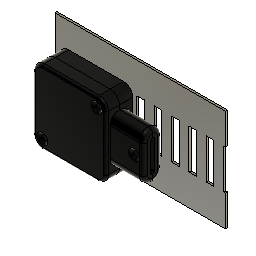
Prog Backpack v22 (Autodesk Fusion 360 design; units mm, degrees)
Autodesk Fusion 360 part; units mm, degrees
sketch "GCP Metal Case" plane through (0, 0, 0) normal (0, 1, 0) x (1, 0, 0)
  line L0 (-58.7401, 16.0721) -> (43.7757, 16.0721) construction
  line L1 (-58.7401, 46.7071) -> (43.7757, 46.7071)
  line L2 (43.7757, -14.5628) -> (-58.7401, -14.5628)
  line L3 (57.6, 4.0721) -> (53.15, 4.0721)
  line L4 (32.25, 4.0721) -> (32.25, 28.0721)
  line L5 (-15.55, 28.0721) -> (-15.55, 4.0721)
  line L6 (-30.45, 16.0721) -> (-26, 16.0721) construction
  line L7 (11.35, 4.0721) -> (11.35, 28.0721)
  line L8 (26.25, 28.0721) -> (26.25, 4.0721)
  line L9 (0.9, 4.0721) -> (0.9, 28.0721)
  line L10 (15.8, 4.0721) -> (11.35, 4.0721)
  line L11 (47.15, 28.0721) -> (47.15, 4.0721)
  line L12 (53.15, 4.0721) -> (53.15, 28.0721)
  line L13 (-9.55, 4.0721) -> (-9.55, 28.0721)
  line L14 (-20, 28.0721) -> (-15.55, 28.0721)
  line L15 (-26, 4.0721) -> (-30.45, 4.0721)
  line L16 (-30.45, 4.0721) -> (-30.45, 28.0721)
  line L17 (21.8, 4.0721) -> (21.8, 28.0721)
  line L18 (5.35, 28.0721) -> (5.35, 4.0721)
  line L19 (-58.7401, -14.5628) -> (-58.7401, 46.7071)
  line L20 (-20, 4.0721) -> (-20, 28.0721)
  line L21 (-5.1, 4.0721) -> (-9.55, 4.0721)
  line L22 (-15.55, 4.0721) -> (-20, 4.0721)
  line L23 (0.9, 28.0721) -> (5.35, 28.0721)
  line L24 (36.7, 28.0721) -> (36.7, 4.0721)
  line L25 (26.25, 4.0721) -> (21.8, 4.0721)
  line L26 (15.8, 28.0721) -> (15.8, 4.0721)
  line L27 (21.8, 28.0721) -> (26.25, 28.0721)
  line L28 (53.15, 28.0721) -> (57.6, 28.0721)
  line L29 (47.15, 4.0721) -> (42.7, 4.0721)
  line L30 (-5.1, 28.0721) -> (-5.1, 4.0721)
  line L31 (-9.55, 28.0721) -> (-5.1, 28.0721)
  line L32 (36.7, 4.0721) -> (32.25, 4.0721)
  line L33 (-30.45, 28.0721) -> (-26, 28.0721)
  line L34 (11.35, 28.0721) -> (15.8, 28.0721)
  line L35 (42.7, 4.0721) -> (42.7, 28.0721)
  line L36 (-26, 28.0721) -> (-26, 4.0721)
  line L37 (5.35, 4.0721) -> (0.9, 4.0721)
  line L38 (43.7757, 46.7071) -> (43.7757, -14.5628)
  line L39 (32.25, 28.0721) -> (36.7, 28.0721)
  line L40 (57.6, 28.0721) -> (57.6, 4.0721)
  line L41 (42.7, 28.0721) -> (47.15, 28.0721)
  dimension "d3" = 10.45
  dimension "d4" = 0
  dimension "d23" = 4.45
  dimension "d24" = 24
  constraint horizontal L1
  constraint vertical L38
  constraint horizontal L2
  constraint vertical L19
  constraint midpoint L0.start L19
  constraint midpoint L0.end L38
  constraint horizontal L33
  constraint vertical L36
  constraint horizontal L15
  constraint vertical L16
  constraint midpoint L6.start L16
  constraint midpoint L6.end L36
  constraint collinear L0 L6
  measures "d23" distance of L16 L36
  measures "d24" distance of L15 L33
extrude "Extrude1" add sketch "GCP Metal Case" along normal blind 1.25 contours L1 L2 L19 L29 L35 L38 L41 makes body 1
sketch "Internals" plane through (0, 0, 0) normal (0, 1, 0) x (1, 0, 0)
  line L0 (-20, 4.0721) -> (-20, 28.0721)
  line L1 (-15.55, 4.0721) -> (-20, 4.0721)
  line L2 (-15.55, 28.0721) -> (-15.55, 4.0721)
  line L3 (-20, 28.0721) -> (-15.55, 28.0721)
  line L4 (-47.05, 3.5721) -> (-31.55, 3.5721)
  line L5 (-31.55, 41.5721) -> (-47.05, 41.5721)
  line L6 (-30.45, 4.0721) -> (-30.45, 28.0721)
  line L7 (-26, 4.0721) -> (-30.45, 4.0721)
  line L8 (-26, 28.0721) -> (-26, 4.0721)
  line L9 (-30.45, 28.0721) -> (-26, 28.0721)
  circle A0 centre (-17.75, 6.2721) radius 1.575
  line L10 (-12.05, 0.5721) -> (-56.05, 0.5721)
  line L11 (-56.05, 0.5721) -> (-56.05, 44.5721)
  line L12 (-26.2, 26.8721) -> (-26.2, 5.2721)
  line L13 (-27.2, 4.2721) -> (-29.25, 4.2721)
  line L14 (-30.25, 5.2721) -> (-30.25, 26.8721)
  line L15 (-29.25, 27.8721) -> (-27.2, 27.8721)
  arc A1 (-30.25, 5.2721) -> (-29.25, 4.2721) centre (-29.25, 5.2721) ccw
  arc A2 (-27.2, 4.2721) -> (-26.2, 5.2721) centre (-27.2, 5.2721) ccw
  arc A3 (-26.2, 26.8721) -> (-27.2, 27.8721) centre (-27.2, 26.8721) ccw
  arc A4 (-29.25, 27.8721) -> (-30.25, 26.8721) centre (-29.25, 26.8721) ccw
  line L16 (-47.05, 3.5721) -> (-47.05, 41.5721)
  line L17 (-31.55, 28.4331) -> (-31.55, 15.5183)
  line L18 (-31.55, 3.5721) -> (-31.55, 15.5183)
  line L19 (-31.55, 28.4331) -> (-31.55, 41.5721)
  line L20 (-9.55, 4.0721) -> (-9.55, 28.0721)
  line L21 (-5.1, 4.0721) -> (-9.55, 4.0721)
  line L22 (-5.1, 28.0721) -> (-5.1, 4.0721)
  line L23 (-9.55, 28.0721) -> (-5.1, 28.0721)
  line L24 (-15.55, 28.0721) -> (-15.55, 4.0721)
  line L25 (-55.05, 33.4471) -> (-41.85, 33.4471)
  line L26 (-41.85, 33.4471) -> (-41.85, 11.6971)
  line L27 (-56.05, 17.9471) -> (-56.05, 27.1971)
  line L28 (-41.85, 11.6971) -> (-55.05, 11.6971)
  line L29 (-56.05, 27.1971) -> (-55.05, 27.1971)
  line L30 (-55.05, 27.1971) -> (-55.05, 17.9471)
  circle A5 centre (-52.55, 14.1971) radius 1.5
  line L31 (-55.05, 11.6971) -> (-55.05, 33.4471)
  circle A6 centre (-52.55, 30.9471) radius 1.5
  line L32 (-55.05, 17.9471) -> (-56.05, 17.9471)
  arc A7 (-27.2, 4.7721) -> (-26.7, 5.2721) centre (-27.2, 5.2721) ccw
  line L33 (-26.7, 26.8721) -> (-26.7, 5.2721)
  arc A8 (-26.7, 26.8721) -> (-27.2, 27.3721) centre (-27.2, 26.8721) ccw
  line L34 (-29.25, 27.3721) -> (-27.2, 27.3721)
  arc A9 (-29.25, 27.3721) -> (-29.75, 26.8721) centre (-29.25, 26.8721) ccw
  line L35 (-29.75, 5.2721) -> (-29.75, 8.2721)
  arc A10 (-29.75, 5.2721) -> (-29.25, 4.7721) centre (-29.25, 5.2721) ccw
  line L36 (-27.2, 4.7721) -> (-29.25, 4.7721)
  arc A11 (-19.8, 5.2721) -> (-18.8, 4.2721) centre (-18.8, 5.2721) ccw
  line L37 (-19.8, 5.2721) -> (-19.8, 26.8721)
  arc A12 (-18.8, 27.8721) -> (-19.8, 26.8721) centre (-18.8, 26.8721) ccw
  line L38 (-18.8, 27.8721) -> (-16.75, 27.8721)
  arc A13 (-15.75, 26.8721) -> (-16.75, 27.8721) centre (-16.75, 26.8721) ccw
  line L39 (-15.75, 26.8721) -> (-15.75, 5.2721)
  arc A14 (-16.75, 4.2721) -> (-15.75, 5.2721) centre (-16.75, 5.2721) ccw
  line L40 (-16.75, 4.2721) -> (-18.8, 4.2721)
  line L41 (-31.55, 8.2721) -> (-29.75, 8.2721)
  line L42 (-29.75, 8.2721) -> (-29.75, 26.8721)
  line L43 (-29.75, 24.3721) -> (-31.55, 24.3721)
  line L44 (-26.7, 8.2721) -> (-15.75, 8.2721)
  line L45 (-26.7, 24.3721) -> (-15.75, 24.3721)
  line L46 (-12.05, 0.5721) -> (-12.05, 44.5721)
  line L47 (-56.05, 44.5721) -> (-12.05, 44.5721)
  circle A15 centre (-50.35, 38.8721) radius 1.575
  line L48 (-47.6, 40.4598) -> (-50.35, 42.0475)
  line L49 (-50.35, 42.0475) -> (-53.1, 40.4598)
  line L50 (-53.1, 40.4598) -> (-53.1, 37.2844)
  line L51 (-53.1, 37.2844) -> (-50.35, 35.6967)
  line L52 (-50.35, 35.6967) -> (-47.6, 37.2844)
  line L53 (-47.6, 37.2844) -> (-47.6, 40.4598)
  point P0 (-50.35, 38.8721)
  dimension "d15" = 15.5
  dimension "d17" = 3.15
  dimension "d19" = 44
  dimension "d20" = 44
  dimension "d21" = 3.5
  dimension "d27" = 1
  dimension "d69" = 5.7
  dimension "d72" = 13.2
  dimension "d73" = 21.75
  dimension "d75" = 9.25
  dimension "d76" = 6.25
  dimension "d77" = 3
  dimension "d78" = 3
  dimension "d79" = 2.5
  dimension "d80" = 2.5
  dimension "d81" = 2.5
  dimension "d82" = 2.5
  dimension "d86" = 1
  dimension "d91" = 11.125
  dimension "d93" = 3
  dimension "d100" = 10.45
  dimension "d101" = 0
  dimension "d104" = 3
  dimension "d105" = 3.5
  dimension "d142" = 5.7
  dimension "d143" = 11.125
  dimension "d144" = 3.15
  dimension "d145" = 5.7
  dimension "d146" = 5.7
  dimension "d147" = 9
  dimension "d148" = 12.05
  dimension "d149" = 3
  dimension "d150" = 2.75
  constraint horizontal L4
  constraint vertical L18
  constraint horizontal L5
  constraint horizontal L10
  constraint vertical L11
  constraint tangent L14 A1
  constraint tangent L13 A1
  constraint tangent L13 A2
  constraint tangent L12 A2
  constraint equal A1 A2
  constraint tangent L12 A3
  constraint tangent L15 A3
  constraint equal A1 A3
  constraint tangent L15 A4
  constraint tangent L14 A4
  constraint equal A1 A4
  constraint perpendicular L5 L16
  constraint vertical L17
  constraint collinear L18 L19
  constraint horizontal L25
  constraint vertical L26
  constraint horizontal L28
  constraint vertical L31
  constraint horizontal L29
  constraint vertical L30
  constraint horizontal L32
  constraint vertical L27
  constraint coincident L30.end L31
  constraint collinear L11 L27
  constraint vertical L42
  constraint coincident L18 L41.start
  constraint concentric A2 A7
  constraint concentric A3 A8
  constraint concentric A4 A9
  constraint concentric A1 A10
  constraint tangent A8 L34
  constraint tangent A7 L36
  constraint tangent L33 A8
  constraint tangent A7 L33
  constraint tangent L34 A9
  constraint tangent L35 A10
  constraint tangent A9 L35
  constraint tangent A10 L36
  constraint coincident L42 L43.start
  constraint coincident L17 L43.end
  constraint perpendicular L17 L43
  constraint coincident L33 L44.start
  constraint coincident L39 L44.end
  constraint perpendicular L39 L44
  constraint coincident L33 L45.start
  constraint coincident L39 L45.end
  constraint perpendicular L39 L45
  constraint collinear L41 L44
  constraint collinear L43 L45
  constraint perpendicular L10 L46
  constraint perpendicular L46 L47
  constraint coincident P0 A15.centre
  measures "d15" distance of L4.start L4.end
  measures "d17" diameter of A0
  measures "d19" distance of L10.end L11.end
  measures "d20" distance of L10.start L10.end
  measures "d21" distance of L7 L10
  measures "d27" radius of A1
  measures "d69" distance of A0.centre L10
  measures "d72" distance of L25.end L25.start
  measures "d73" distance of L25.start L28.end
  measures "d75" distance of L27.start L27.end
  measures "d76" distance of L25 L29
  measures "d77" diameter of A6
  measures "d78" diameter of A5
  measures "d79" distance of A6.centre L31
  measures "d80" distance of A6.centre L25
  measures "d81" distance of A5.centre L31
  measures "d82" distance of A5.centre L28
  measures "d86" distance of L29.end L27.end
  measures "d91" distance of L10 L28
  measures "d93" distance of L4 L10
  measures "d104" distance of L34 L43
  measures "d105" distance of L36 L41
  measures "d142" distance of A0.centre L46
  measures "d143" distance of L25 L47
  measures "d144" diameter of A15
  measures "d145" distance of L11 P0
  measures "d146" distance of L47 P0
  measures "d147" distance of L11 L16
  measures "d148" distance of origin L46
  measures "d149" distance of L5 L47
  measures "d150" distance of P0 L53
extrude "Extrude2" add sketch "Internals" against normal blind 1 separate body contours L0 L1 L2 L3 L4 L5 L6 L7 L8 L9 L10 L11 L16 L17 L18 L19 L24 L25 L28 L29 L31 L32 L41 L43 L44 L45 L46 L47 | L0 L1 L2 L3 L24 A11 L37 A12 L38 A13 L39 A14 L40 L44 L45 | L0 L8 L44 L45 | L0 L37 L44 L45 | L8 L12 L44 L45 | L6 L7 L8 L12 L13 L14 A1 A2 L41 L44 | A11 L37 L39 A14 L40 L44 | L37 L39 L44 L45 | L6 L8 L9 L12 L14 L15 A3 A4 L43 L45 | L37 A12 L38 A13 L39 L45 | L12 L33 L44 L45 | L12 L13 L14 A1 A2 A7 L33 L35 A10 L36 L41 L44 | L12 L14 L15 A3 A4 L33 A8 L34 A9 L42 L43 L45 | L6 L17 L18 L41 L43 | L6 L14 L41 L43 | L4 L5 L16 L17 L18 L19 L25 L26 L28 | L14 L41 L42 L43 | L16 L25 L28 L30 L31 | L16 L25 L26 L28 | L11 L27 L29 L30 L31 L32 | A5 | A6 | L48 L49 L50 L51 L52 L53 makes body 2
extrude "Extrude3" add sketch "Internals" against normal blind 8 contours L0 L1 L2 L3 L4 L5 L6 L7 L8 L9 L10 L11 L16 L17 L18 L19 L24 L25 L28 L29 L31 L32 L41 L43 L44 L45 L46 L47 | L0 L1 L2 L3 L24 A11 L37 A12 L38 A13 L39 A14 L40 L44 L45 | L0 L8 L44 L45 | L0 L37 L44 L45 | L8 L12 L44 L45 | L6 L7 L8 L12 L13 L14 A1 A2 L41 L44 | A11 L37 L39 A14 L40 L44 | L37 L39 L44 L45 | L6 L8 L9 L12 L14 L15 A3 A4 L43 L45 | L37 A12 L38 A13 L39 L45 | L12 L33 L44 L45 | L12 L13 L14 A1 A2 A7 L33 L35 A10 L36 L41 L44 | L12 L14 L15 A3 A4 L33 A8 L34 A9 L42 L43 L45 | L6 L17 L18 L41 L43 | L6 L14 L41 L43 | L14 L41 L42 L43 | L16 L25 L28 L30 L31 | L11 L27 L29 L30 L31 L32 | A5 | A6 | L48 L49 L50 L51 L52 L53 bodies 2
extrude "Extrude10" add sketch "Internals" along normal blind 1 contours A11 L37 L39 A14 L40 L44 | L37 L39 L44 L45 | L37 A12 L38 A13 L39 L45 | L12 L33 L44 L45 | L12 L13 L14 A1 A2 A7 L33 L35 A10 L36 L41 L44 | L12 L14 L15 A3 A4 L33 A8 L34 A9 L42 L43 L45 | L14 L41 L42 L43 bodies 2
extrude "Extrude11" add sketch "Internals" against normal blind 6 from surface at -8 separate body contours L0 L1 L2 L3 L4 L5 L6 L7 L8 L9 L10 L11 L16 L17 L18 L19 L24 L25 L28 L29 L31 L32 L41 L43 L44 L45 L46 L47 | L0 L1 L2 L3 L24 A11 L37 A12 L38 A13 L39 A14 L40 L44 L45 | L0 L8 L44 L45 | L0 L37 L44 L45 | L8 L12 L44 L45 | L6 L7 L8 L12 L13 L14 A1 A2 L41 L44 | A11 L37 L39 A14 L40 L44 | L37 L39 L44 L45 | L6 L8 L9 L12 L14 L15 A3 A4 L43 L45 | L37 A12 L38 A13 L39 L45 | L12 L33 L44 L45 | L12 L13 L14 A1 A2 A7 L33 L35 A10 L36 L41 L44 | L12 L14 L15 A3 A4 L33 A8 L34 A9 L42 L43 L45 | A7 L33 A8 L34 A9 L35 A10 L36 L42 | L6 L17 L18 L41 L43 | L6 L14 L41 L43 | L14 L41 L42 L43 | A5 | A6 | L48 L49 L50 L51 L52 L53 makes body 3 at (-52.1437, -12, -15.6411) makes body 4 at (-53.2343, -12, -29.6123) makes body 5 at (-20.3332, -8, -26.9376)
extrude "Extrude12" add sketch "Internals" against normal blind 2 from surface at -14 contours L0 L1 L2 L3 L4 L5 L6 L7 L8 L9 L10 L11 L16 L17 L18 L19 L24 L25 L28 L29 L31 L32 L41 L43 L44 L45 L46 L47 | L0 L1 L2 L3 L24 A11 L37 A12 L38 A13 L39 A14 L40 L44 L45 | L0 L8 L44 L45 | L0 L37 L44 L45 | L8 L12 L44 L45 | L6 L7 L8 L12 L13 L14 A1 A2 L41 L44 | A11 L37 L39 A14 L40 L44 | L37 L39 L44 L45 | L6 L8 L9 L12 L14 L15 A3 A4 L43 L45 | L37 A12 L38 A13 L39 L45 | L12 L33 L44 L45 | L12 L13 L14 A1 A2 A7 L33 L35 A10 L36 L41 L44 | L12 L14 L15 A3 A4 L33 A8 L34 A9 L42 L43 L45 | A7 L33 A8 L34 A9 L35 A10 L36 L42 | L6 L17 L18 L41 L43 | L6 L14 L41 L43 | L4 L5 L16 L17 L18 L19 L25 L26 L28 | L14 L41 L42 L43 | L16 L25 L28 L30 L31 | L16 L25 L26 L28 | L11 L27 L29 L30 L31 L32 | A5 | A6 | L48 L49 L50 L51 L52 L53 bodies 3 4 5
sketch "Pogo" plane through (0, 0, 0) normal (1, 0, 0) x (0, 1, 0)
  line L0 (-12.125, -14.0721) -> (-12.125, -31.0721)
  arc A0 (-12.125, -31.0721) -> (-3.875, -31.0721) centre (-8, -31.0721) ccw
  line L1 (-3.875, -31.0721) -> (-3.875, -14.0721)
  arc A1 (-3.875, -14.0721) -> (-12.125, -14.0721) centre (-8, -14.0721) ccw
  line L2 (-11.125, -14.0721) -> (-11.125, -31.0721)
  arc A2 (-11.125, -31.0721) -> (-4.875, -31.0721) centre (-8, -31.0721) ccw
  arc A3 (-4.875, -14.0721) -> (-11.125, -14.0721) centre (-8, -14.0721) ccw
  line L3 (-4.875, -31.0721) -> (-4.875, -14.0721)
  line L4 (-16, -0.5721) -> (-16, -44.5721)
  line L5 (0, -44.5721) -> (0, -0.5721)
  line L6 (-9, -0.5721) -> (-16, -0.5721)
  line L7 (-1.4, -44.5721) -> (-16, -44.5721)
  dimension "d123" = 3.875
  dimension "d124" = 3.875
  dimension "d125" = 8.25
  dimension "d126" = 6.25
  dimension "d128" = 17
  dimension "d129" = 17
  dimension "d130" = 1
  dimension "d131" = 1
  dimension "d132" = 13.5
  dimension "d133" = 13.5
  dimension "d134" = 17
  dimension "d186" = 16
  constraint parallel L2 L3
  constraint tangent L2 A2
  constraint tangent A2 L3
  constraint tangent L2 A3
  constraint tangent A3 L3
  constraint parallel L0 L1
  constraint tangent L0 A0
  constraint tangent A0 L1
  constraint tangent L0 A1
  constraint tangent L1 A1
  constraint perpendicular L4 L6
  constraint perpendicular L4 L7
  constraint horizontal L6
  measures "d123" distance of L0 L4
  measures "d124" distance of L1 L5
  measures "d125" distance of L0 L1
  measures "d126" distance of L2 L3
  measures "d128" distance of L0.start L0.end
  measures "d129" distance of L2.start L2.end
  measures "d130" distance of L0 L2
  measures "d131" distance of L1 L3
  measures "d132" distance of A1.centre L6
  measures "d133" distance of A0.centre L7
  measures "d134" distance of A0.centre A1.centre
  measures "d186" distance of L4 L5.end
extrude "Extrude17" cut sketch "Pogo" against normal blind 36 contours L2 A2 A3 L3 bodies 2 3
extrude "Extrude18" cut sketch "Pogo" against normal blind 1 from surface at -13.3 bodies 2 3
chamfer "Chamfer3" distance 1.75 angle 45 2 edges at (-19.2184, -16, -5.7026) (-51.8184, -16, -38.3026) on bodies 3
extrude "Extrude19" cut sketch "Internals" against normal blind 4 contours L48 L49 L50 L51 L52 L53 bodies 2
fillet "Fillet1" radius 5.5 8 edges at (-56.05, -12, -44.5721) (-12.05, -12, -44.5721) (-56.05, -12, -0.5721) (-12.05, -12, -0.5721) (-56.05, -4, -44.5721) (-12.05, -4, -44.5721) (-56.05, -4, -0.5721) (-12.05, -4, -0.5721) on bodies 2 3
fillet "Fillet2" radius 1.5 8 edges at (-13.6609, -16, -42.9612) (-12.05, -16, -22.5721) (-13.6609, -16, -2.183) (-34.05, -16, -0.5721) (-54.4391, -16, -2.183) (-56.05, -16, -22.5721) (-54.4391, -16, -42.9612) (-34.05, -16, -44.5721) on bodies 3
sketch "usb c cleanup" plane through (0, -14, 0) normal (0, 1, 0) x (-1, 0, 0)
  line L0 (56.05, -17.9471) -> (55.05, -17.9471)
  line L1 (55.05, -17.9471) -> (55.05, -11.6971)
  line L2 (55.05, -11.6971) -> (47.05, -11.6971)
  line L3 (47.05, -11.6971) -> (47.05, -3.5721)
  line L4 (47.05, -3.5721) -> (31.55, -3.5721)
  line L5 (31.55, -3.5721) -> (31.55, -41.5721)
  line L6 (31.55, -41.5721) -> (47.05, -41.5721)
  line L7 (47.05, -41.5721) -> (47.05, -33.4471)
  line L8 (47.05, -33.4471) -> (55.05, -33.4471)
  line L9 (55.05, -33.4471) -> (55.05, -27.1971)
  line L10 (55.05, -27.1971) -> (56.05, -27.1971)
  line L11 (56.05, -27.1971) -> (56.05, -17.9471)
  circle A0 centre (52.55, -14.1971) radius 1.5
  circle A1 centre (52.55, -30.9471) radius 1.5
  line L12 (56.05, -27.1971) -> (55.05, -27.1971)
  line L13 (55.05, -27.1971) -> (55.05, -17.9471)
  line L14 (55.05, -17.9471) -> (56.05, -17.9471)
  line L15 (56.05, -17.9471) -> (56.05, -27.1971)
  constraint horizontal L12
  constraint vertical L13
  constraint horizontal L14
  constraint vertical L15
  constraint coincident L0.end L1.start
  constraint coincident L10.end L11.start
extrude "Extrude20" add sketch "usb c cleanup" along normal blind 2 contours L0 L10 L11 L12 L13 L14 L15 bodies 3
fillet "Fillet3" radius 0.5 2 edges at (-55.55, -12, -27.1971) (-55.55, -12, -17.9471) on bodies 3
sketch "pcb holders" plane through (0, 0, -3.5721) normal (0, 0, -1) x (1, 0, 0)
  line L0 (-31.55, 1) -> (-31.55, 8)
  line L1 (-31.55, 8) -> (-47.05, 8)
  line L2 (-47.05, 8) -> (-47.05, 1)
  line L3 (-47.05, 4) -> (-46.05, 4)
  line L4 (-47.05, 6) -> (-47.05, 4)
  line L5 (-46.05, 4) -> (-47.05, 6)
  line L6 (-31.55, 4) -> (-32.55, 4)
  line L7 (-32.55, 4) -> (-32.55, 6)
  line L8 (-32.55, 6) -> (-31.55, 6)
  line L9 (-31.55, 6) -> (-31.55, 4)
  line L10 (-32.55, 4) -> (-31.55, 6)
  line L11 (-47.05, 1) -> (-31.55, 1)
  dimension "d166" = 1
  dimension "d167" = 2
  dimension "d170" = 1
  dimension "d171" = 2
  constraint horizontal L3
  constraint vertical L4
  constraint coincident L2 L3.start
  constraint horizontal L6
  constraint vertical L7
  constraint horizontal L8
  constraint vertical L9
  constraint coincident L0 L6.start
  measures "d166" distance of L3.start L3.end
  measures "d167" distance of L3.start L4.start
  measures "d170" distance of L6.start L6.end
  measures "d171" distance of L6.start L8.end
extrude "Extrude21" add sketch "pcb holders" along normal blind 40 contours L2 L3 L4 L5 bodies 2
extrude "Extrude22" add sketch "pcb holders" along normal blind 6.5 contours L0 L6 L9 L10 bodies 2
sketch "plug" plane through (0, 0, 0) normal (0, 1, 0) x (1, 0, 0)
  line L0 (-12, 7) -> (8, 7)
  line L1 (8, 7) -> (8, 37)
  line L2 (8, 37) -> (-12, 37)
  line L3 (-12, 37) -> (-12, 7)
  dimension "d175" = 30
  dimension "d176" = 7
  dimension "d190" = 20
  constraint horizontal L0
  constraint vertical L1
  constraint horizontal L2
  constraint vertical L3
  measures "d175" distance of L0.start L2.end
  measures "d176" distance of origin L0
  measures "d190" distance of L1 L3
extrude "Extrude23" add sketch "plug" against normal blind 5.825 from surface at -2.175 separate body makes body 6
extrude "Extrude24" add sketch "plug" against normal blind 5.825 from surface at -8 separate body makes body 7
extrude "Extrude25" cut sketch "Pogo" against normal blind 7.5 from surface at -4.5 contours L2 A2 A3 L3 bodies 6 7
extrude "Extrude26" cut sketch "Pogo" along normal blind 1.25 from surface at -11.2 bodies 6 7
sketch "wire hole" plane through (0, 0, 0) normal (1, 0, 0) x (0, 1, 0)
  arc A0 (-3.875, -14.0721) -> (-12.125, -14.0721) centre (-8, -14.0721) ccw
  line L0 (-12.125, -14.0721) -> (-12.125, -31.0721)
  line L1 (-3.875, -31.0721) -> (-3.875, -14.0721)
  arc A1 (-12.125, -31.0721) -> (-3.875, -31.0721) centre (-8, -31.0721) ccw
  arc A2 (-2.375, -14.0721) -> (-13.625, -14.0721) centre (-8, -14.0721) ccw
  line L2 (-13.625, -14.0721) -> (-13.625, -31.0721)
  arc A3 (-13.625, -31.0721) -> (-2.375, -31.0721) centre (-8, -31.0721) ccw
  line L3 (-2.375, -31.0721) -> (-2.375, -14.0721)
  line L4 (-6.875, -31.0721) -> (-6.875, -14.0721)
  arc A4 (-6.875, -14.0721) -> (-9.125, -14.0721) centre (-8, -14.0721) ccw
  line L5 (-9.125, -14.0721) -> (-9.125, -31.0721)
  arc A5 (-9.125, -31.0721) -> (-6.875, -31.0721) centre (-8, -31.0721) ccw
  line L6 (2.3949, -4.3818) -> (-18.4184, -4.3818)
  line L7 (-18.4184, -4.3818) -> (-18.4184, -40.7624)
  line L8 (-18.4184, -40.7624) -> (2.3949, -40.7624)
  line L9 (2.3949, -40.7624) -> (2.3949, -4.3818)
  line L10 (2.3949, -4.3818) -> (-18.4184, -40.7624) construction
  line L11 (-18.4184, -4.3818) -> (2.3949, -40.7624) construction
  point P0 (-8.0118, -22.5721)
  dimension "d191" = 1.5
  dimension "d192" = -3
  constraint horizontal L6
  constraint perpendicular L6 L7
  constraint parallel L6 L8
  constraint parallel L7 L9
  constraint coincident L10 P0
  constraint coincident L11 P0
extrude "Extrude27" cut sketch "wire hole" along normal mid plane 32 contours L4 A4 L5 A5 bodies 6 7
extrude "Extrude28" cut sketch "wire hole" along normal mid plane 30 contours L6 L7 L8 L9 bodies 6 7
fillet "Fillet5" radius 2.5 6 edges at (8, -4.0225, -35.0496) (8, -2.375, -22.5721) (8, -4.0225, -10.0946) (8, -11.9775, -10.0946) (8, -13.625, -22.5721) (8, -11.9775, -35.0496) on bodies 6 7
sketch "plug bolt" plane through (0, 0, 0) normal (0, 1, 0) x (1, 0, 0)
  circle A0 centre (2.5, 22) radius 1.55
  line L0 (5.2499, 23.5878) -> (2.4999, 25.1754)
  line L1 (2.4999, 25.1754) -> (-0.2501, 23.5876)
  line L2 (-0.2501, 23.5876) -> (-0.2499, 20.4122)
  line L3 (-0.2499, 20.4122) -> (2.5001, 18.8246)
  line L4 (2.5001, 18.8246) -> (5.2501, 20.4124)
  line L5 (5.2501, 20.4124) -> (5.2499, 23.5878)
  line L6 (-12, 14.0721) -> (-12, 31.0721)
  point P0 (2.5, 22)
  dimension "d200" = 3.1
  dimension "d201" = 2.75
  dimension "d209" = 14.5
  constraint coincident P0 A0.centre
  measures "d200" diameter of A0
  measures "d201" distance of P0 L5
  measures "d209" distance of P0 L6
extrude "Extrude29" cut sketch "plug bolt" against normal blind 25 contours A0 bodies 6 7
extrude "Extrude30" cut sketch "plug bolt" against normal blind 2 from surface at -2.375 bodies 6
chamfer "Chamfer4" distance 1.75 angle 45 1 edges at (1.0549, -13.625, -21.4395) on bodies 7
equation "d23 = slotWidth"
equation "d24 = slotHeight"
equation "slotWidth = 4.45 mm" comment "GCP Slot width"
equation "slotHeight = 24 mm" comment "GCP Slot height"
equation "slotThick = 1.25 mm" comment "GCP Slot thick"
equation "slotSpacing = 10.45 mm" comment "GCP Slot Spacing"
equation "d11 = slotThick"
equation "d41 = 21.75 mm"
equation "d45 = 9.25 mm"
equation "d49 = 2.5 mm"
equation "d76 = ( d41 - d45 ) / 2"
equation "d80 = d49"
equation "d81 = d49"
equation "d82 = d49"
equation "d100 = slotSpacing"
equation "d129 = d128"
equation "d134 = d128"
equation "d150 = ( 5.5 / 2 ) * 1 mm"
equation "d176 = ( ( 44 - 30 ) / 2 ) * 1 mm"
equation "d178 = -8 mm + 2.175 mm"
equation "d201 = ( 5.5 / 2 ) * 1 mm"
named bodies: "metal housing", "BP top", "BP bottom", "Plug bottom", "Plug top"
